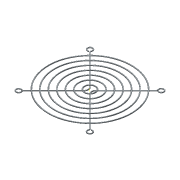
# Autodesk Inventor part: Fan Guard
Saved by Autodesk Inventor 2017 (Build 210142000, 142)
## iProperties
Created: 2008-03-24
Part Number: Fan Guard
Document SubType Name: Modeling
Designer: Administrator
Density: 1 g/cm^3
Mass: 3.71299 g
Surface Area: 93.6347 cm^2
Volume: 3.71299 cm^3
Material: Generic
Appearance: Zinc
Author: Administrator
Autodesk Inventor part; units mm, degrees
sketch "Sketch1" plane through (0, 0, 0) normal (0, 0, 1) x (1, 0, 0)
  circle A0 centre (7.9375, 0) radius 0.7937
  circle A1 centre (16.7821, 0) radius 0.7937
  circle A2 centre (25.6268, 0) radius 0.7937
  circle A3 centre (34.4714, 0) radius 0.7937
  circle A4 centre (43.3161, 0) radius 0.7937
  circle A5 centre (52.1607, 0) radius 0.7937
  circle A6 centre (61.0054, 0) radius 0.7937
  circle A7 centre (69.85, 0) radius 0.7937
  line L0 (7.9375, 0) -> (16.7821, 0) construction
  line L1 (16.7821, 0) -> (25.6268, 0) construction
  line L2 (25.6268, 0) -> (34.4714, 0) construction
  line L3 (34.4714, 0) -> (43.3161, 0) construction
  line L4 (43.3161, 0) -> (52.1607, 0) construction
  line L5 (52.1607, 0) -> (61.0054, 0) construction
  line L6 (61.0054, 0) -> (69.85, 0) construction
  line L7 (0, -1.1113) -> (0, 1.1113) projected
  point P0 (0, 0)
  dimension "d0" = 1.5875
  dimension "d1" = 139.7
  dimension "d2" = 15.875
  constraints: 14 end point, 8 centre point, 7 equal radius, 7 horizontal, 6 collinear, 1 horizontal alignment
  measures "d0" diameter of A0
  measures "d1" diameter of L6.end L7
  measures "d2" diameter of L0.start L7
revolve "Revolution1" add sketch "Sketch1" angle 360 about axis through (0, -10, 0) along (0, 1, 0) contours A0 | A1 | A2 | A3 | A4 | A5 | A6
ref_plane "Work Plane1" through (0, -1.5875, 0) normal (0, 1, 0) x (-1, 0, 0)
sketch "Sketch2" plane through (0, -1.5875, 0) normal (0, 1, 0) x (-1, 0, 0)
  line L0 (48.6946, 48.7849) -> (4.3999, 4.4901)
  arc A0 (4.3999, 4.4901) -> (2.54, 0) centre (8.89, 0) ccw
  arc A1 (48.6946, 48.7849) -> (49.1179, 51.0398) centre (47.2578, 50.2217) ccw
  arc A2 (50.878, 49.2405) -> (49.1179, 51.0398) centre (52.3875, 52.4778) ccw
  line L1 (0, -11.5058) -> (0, 69.0346) projected
  line L2 (52.3875, 52.4778) -> (50.878, 49.2405) construction
  point P0 (0, 0)
  dimension "d6" = 7.1437
  dimension "d7" = 2.032
  dimension "d8" = 45
  dimension "d9" = 6.35
  dimension "d10" = 2.54
  dimension "d11" = 20
  dimension "d14" = 52.3875
  constraints: 6 point on circle, 4 end point, 3 centre point, 3 tangent, 2 horizontal alignment, 1 point on line
  measures "d6" diameter of A2
  measures "d7" radius of A1
  measures "d8" angle of L1 L0
  measures "d9" radius of A0
  measures "d10" distance from line of A0.end L1
  measures "d11" angle of L2 L0
  measures "d14" distance from line of L2.start L1
ref_plane "Work Plane2" through (-2.54, -1.5875, 0) normal (0, 0, 1) x (1, 0, 0)
sketch "Sketch3" plane through (-2.54, -1.5875, 0) normal (0, 0, 1) x (1, 0, 0)
  line L0 (0, 0) -> (-1.8599, 0) projected
  circle A0 centre (0, 0) radius 0.7937
  point P0 (2.54, 1.5875)
  dimension "d12" = 1.5875
  constraints: 1 centre point, 1 coincident
  measures "d12" diameter of A0
sweep "Sweep1" add profiles "Sketch3" path "Sketch2" path curves A0 L0 A1 A2
mirror "Mirror1" about plane through (0, 0, 0) normal (0, 0, 1) of "Sweep1"
mirror "Mirror2" about plane through (0, 0, 0) normal (1, 0, 0) of "Sweep1", "Mirror1"
ref_plane "Work Plane4" through (-4.3999, -2.3812, 4.4901) normal (0, 1, 0) x (-1, 0, 0)
body "Solid1"
